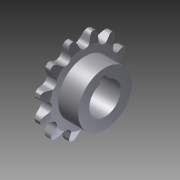
# Autodesk Inventor part: 12t #25 sprocket
Saved by Autodesk Inventor 2012 (Build 160160000, 160)
## iProperties
Created: 2013-07-14
Part Number: 12t #25 sprocket
Material: Default
Document SubType Name: Modeling
Designer: Bryce
Density: 1 g/cm^3
Author: Bryce
Autodesk Inventor part; units mm, degrees
ref_plane "YZ Plane" through (0, 0, 0) normal (1, 0, 0) x (0, 1, 0)
ref_plane "XZ Plane" through (0, 0, 0) normal (0, 1, 0) x (-1, 0, 0)
ref_plane "XY Plane" through (0, 0, 0) normal (0, 0, 1) x (1, 0, 0)
sketch "Sketch1" plane through (0, 0, 0) normal (0, 0, 1) x (1, 0, 0)
  line L0 (0, 0) -> (3.175, 0)
  line L1 (3.175, 0) -> (3.175, 6.1227)
  line L2 (3.175, 8.97) -> (2.4121, 8.97) construction
  line L3 (0, 8.97) -> (0, 6.1227) construction
  line L4 (3.175, 0) -> (9.525, 0)
  line L5 (9.525, 0) -> (9.525, 3.5)
  line L6 (9.525, 3.5) -> (3.175, 3.5)
  line L7 (3.175, 3.5) -> (3.175, 0)
  line L8 (0, -5) -> (9.525, -5) construction
  line L9 (0.7629, 8.97) -> (0, 6.1227)
  line L10 (2.4121, 8.97) -> (3.175, 6.1227)
  line L11 (0.7629, 8.97) -> (0, 8.97) construction
  line L12 (2.4121, 8.97) -> (0.7629, 8.97)
  line L13 (0, 6.1227) -> (0, 0)
  line L14 (3.175, 6.1227) -> (3.175, 8.97) construction
  dimension "d0" = 3.175
  dimension "d1" = 5
  dimension "d3" = 13.97
  dimension "d4" = 8.5
  dimension "d12" = 6.35
  dimension "d26" = 30
  dimension "d27" = 1.6491
  constraints: 30 end point, 9 parallel, 4 perpendicular, 2 horizontal, 1 collinear, 1 horizontal alignment, 1 vertical alignment
  measures "d0" distance of L0.start L0.end
  measures "d1" distance between parallel lines of L4 L8
  measures "d3" distance between parallel lines of L2 L8
  measures "d4" distance between parallel lines of L8 L6
  measures "d12" distance of L0.end L4.end
  measures "d26" angle of L10 L9
  measures "d27" distance of L2.end L9.start
revolve "Revolution1" add sketch "Sketch1" angle 360 about axis through (0, -5, 0) along (1, 0, 0)
sketch "Sketch3" plane through (0, -5, 0) normal (-1, 0, 0) x (0, 0, 1)
  circle A0 centre (0, 0) radius 11.1227 projected
  arc A1 (4.5327, 11.9915) -> (4.0726, 13.3632) centre (2.8057, 12.1753) ccw
  arc A2 (3.1546, 13.6092) -> (2.0703, 12.6513) centre (3.6578, 11.947) ccw
  line L0 (4.4067, 10.8076) -> (4.5327, 11.9915)
  line L1 (1.5875, 11.5629) -> (2.0703, 12.6513)
  arc A3 (-1.5875, 11.5629) -> (1.5875, 11.5629) centre (0, 12.2673) ccw
  line L2 (-1.5875, 11.5629) -> (-2.0703, 12.6513)
  arc A4 (3.1546, 13.6092) -> (-3.1546, 13.6092) centre (0, 0) ccw construction
  arc A5 (-2.0703, 12.6513) -> (-3.1546, 13.6092) centre (-3.6578, 11.947) ccw
  circle A6 centre (0, 0) radius 13.97
  arc A7 (4.0726, 13.3632) -> (3.1546, 13.6092) centre (0, 0) ccw
  arc A8 (-3.1546, 13.6092) -> (-4.0726, 13.3632) centre (0, 0) ccw
  line L3 (-4.4067, 10.8076) -> (-4.5327, 11.9915)
  arc A9 (-4.0726, 13.3632) -> (-4.5327, 11.9915) centre (-2.8057, 12.1753) ccw
  arc A10 (-7.1563, 9.2201) -> (-4.4067, 10.8076) centre (-6.1336, 10.6238) ccw
  arc A11 (-4.0726, 13.3632) -> (-9.5365, 10.2086) centre (0, 0) ccw construction
  line L4 (-7.1563, 9.2201) -> (-8.1186, 9.9211)
  arc A12 (-8.1186, 9.9211) -> (-9.5365, 10.2086) centre (-9.1413, 8.5174) ccw
  arc A13 (-9.5365, 10.2086) -> (-10.2086, 9.5365) centre (0, 0) ccw
  arc A14 (-10.2086, 9.5365) -> (-9.9211, 8.1186) centre (-8.5174, 9.1413) ccw
  arc A15 (-10.8076, 4.4067) -> (-9.2201, 7.1563) centre (-10.6238, 6.1336) ccw
  line L5 (-10.8076, 4.4067) -> (-11.9915, 4.5327)
  arc A16 (-10.2086, 9.5365) -> (-13.3632, 4.0726) centre (0, 0) ccw construction
  arc A17 (-11.9915, 4.5327) -> (-13.3632, 4.0726) centre (-12.1753, 2.8057) ccw
  arc A18 (-13.3632, 4.0726) -> (-13.6092, 3.1546) centre (0, 0) ccw
  line L6 (-9.2201, 7.1563) -> (-9.9211, 8.1186)
  line L7 (-4.4067, -10.8076) -> (-4.5327, -11.9915)
  arc A19 (-4.5327, -11.9915) -> (-4.0726, -13.3632) centre (-2.8057, -12.1753) ccw
  arc A20 (-4.0726, -13.3632) -> (-3.1546, -13.6092) centre (0, 0) ccw
  arc A21 (-9.5365, -10.2086) -> (-4.0726, -13.3632) centre (0, 0) ccw construction
  arc A22 (4.0726, -13.3632) -> (9.5365, -10.2086) centre (0, 0) ccw construction
  arc A23 (7.1563, -9.2201) -> (4.4067, -10.8076) centre (6.1336, -10.6238) ccw
  line L8 (7.1563, -9.2201) -> (8.1186, -9.9211)
  arc A24 (8.1186, -9.9211) -> (9.5365, -10.2086) centre (9.1413, -8.5174) ccw
  arc A25 (9.5365, -10.2086) -> (10.2086, -9.5365) centre (0, 0) ccw
  arc A26 (10.2086, -9.5365) -> (9.9211, -8.1186) centre (8.5174, -9.1413) ccw
  line L9 (9.2201, -7.1563) -> (9.9211, -8.1186)
  arc A27 (10.8076, -4.4067) -> (9.2201, -7.1563) centre (10.6238, -6.1336) ccw
  arc A28 (10.2086, -9.5365) -> (13.3632, -4.0726) centre (0, 0) ccw construction
  arc A29 (11.9915, -4.5327) -> (13.3632, -4.0726) centre (12.1753, -2.8057) ccw
  line L10 (10.8076, -4.4067) -> (11.9915, -4.5327)
  arc A30 (-9.5365, -10.2086) -> (-8.1186, -9.9211) centre (-9.1413, -8.5174) ccw
  line L11 (-7.1563, -9.2201) -> (-8.1186, -9.9211)
  arc A31 (-10.2086, -9.5365) -> (-9.5365, -10.2086) centre (0, 0) ccw
  arc A32 (-9.9211, -8.1186) -> (-10.2086, -9.5365) centre (-8.5174, -9.1413) ccw
  line L12 (-9.2201, -7.1563) -> (-9.9211, -8.1186)
  arc A33 (-9.2201, -7.1563) -> (-10.8076, -4.4067) centre (-10.6238, -6.1336) ccw
  line L13 (-10.8076, -4.4067) -> (-11.9915, -4.5327)
  arc A34 (-13.3632, -4.0726) -> (-11.9915, -4.5327) centre (-12.1753, -2.8057) ccw
  arc A35 (-13.3632, -4.0726) -> (-10.2086, -9.5365) centre (0, 0) ccw construction
  arc A36 (-13.6092, -3.1546) -> (-13.3632, -4.0726) centre (0, 0) ccw
  arc A37 (-4.4067, -10.8076) -> (-7.1563, -9.2201) centre (-6.1336, -10.6238) ccw
  arc A38 (11.5629, 1.5875) -> (11.5629, -1.5875) centre (12.2673, 0) ccw
  line L14 (11.5629, 1.5875) -> (12.6513, 2.0703)
  arc A39 (12.6513, 2.0703) -> (13.6092, 3.1546) centre (11.947, 3.6578) ccw
  line L15 (10.8076, 4.4067) -> (11.9915, 4.5327)
  arc A40 (13.3632, 4.0726) -> (11.9915, 4.5327) centre (12.1753, 2.8057) ccw
  arc A41 (13.6092, 3.1546) -> (13.3632, 4.0726) centre (0, 0) ccw
  line L16 (11.5629, -1.5875) -> (12.6513, -2.0703)
  arc A42 (13.6092, -3.1546) -> (12.6513, -2.0703) centre (11.947, -3.6578) ccw
  arc A43 (13.6092, -3.1546) -> (13.6092, 3.1546) centre (0, 0) ccw construction
  arc A44 (13.3632, -4.0726) -> (13.6092, -3.1546) centre (0, 0) ccw
  arc A45 (9.2201, 7.1563) -> (10.8076, 4.4067) centre (10.6238, 6.1336) ccw
  arc A46 (13.3632, 4.0726) -> (10.2086, 9.5365) centre (0, 0) ccw construction
  line L17 (9.2201, 7.1563) -> (9.9211, 8.1186)
  arc A47 (9.9211, 8.1186) -> (10.2086, 9.5365) centre (8.5174, 9.1413) ccw
  arc A48 (10.2086, 9.5365) -> (9.5365, 10.2086) centre (0, 0) ccw
  arc A49 (9.5365, 10.2086) -> (8.1186, 9.9211) centre (9.1413, 8.5174) ccw
  line L18 (7.1563, 9.2201) -> (8.1186, 9.9211)
  arc A50 (4.4067, 10.8076) -> (7.1563, 9.2201) centre (6.1336, 10.6238) ccw
  arc A51 (9.5365, 10.2086) -> (4.0726, 13.3632) centre (0, 0) ccw construction
  arc A52 (1.5875, -11.5629) -> (-1.5875, -11.5629) centre (0, -12.2673) ccw
  line L19 (1.5875, -11.5629) -> (2.0703, -12.6513)
  arc A53 (2.0703, -12.6513) -> (3.1546, -13.6092) centre (3.6578, -11.947) ccw
  line L20 (-1.5875, -11.5629) -> (-2.0703, -12.6513)
  line L21 (4.4067, -10.8076) -> (4.5327, -11.9915)
  arc A54 (3.1546, -13.6092) -> (4.0726, -13.3632) centre (0, 0) ccw
  arc A55 (-3.1546, -13.6092) -> (-2.0703, -12.6513) centre (-3.6578, -11.947) ccw
  arc A56 (-3.1546, -13.6092) -> (3.1546, -13.6092) centre (0, 0) ccw construction
  arc A57 (4.0726, -13.3632) -> (4.5327, -11.9915) centre (2.8057, -12.1753) ccw
  line L22 (-11.5629, 1.5875) -> (-12.6513, 2.0703)
  arc A58 (-11.5629, -1.5875) -> (-11.5629, 1.5875) centre (-12.2673, 0) ccw
  line L23 (-11.5629, -1.5875) -> (-12.6513, -2.0703)
  arc A59 (-12.6513, -2.0703) -> (-13.6092, -3.1546) centre (-11.947, -3.6578) ccw
  arc A60 (-13.6092, 3.1546) -> (-13.6092, -3.1546) centre (0, 0) ccw construction
  arc A61 (-13.6092, 3.1546) -> (-12.6513, 2.0703) centre (-11.947, 3.6578) ccw
  arc A62 (-4.4511, 10.1932) -> (-6.602, 8.9514) centre (0, 0) ccw
  arc A63 (1.2418, 11.0532) -> (-1.2418, 11.0532) centre (0, 0) ccw
  arc A64 (6.602, 8.9514) -> (4.4511, 10.1932) centre (0, 0) ccw
  arc A65 (10.1932, 4.4511) -> (8.9514, 6.602) centre (0, 0) ccw
  arc A66 (11.0532, -1.2418) -> (11.0532, 1.2418) centre (0, 0) ccw
  arc A67 (8.9514, -6.602) -> (10.1932, -4.4511) centre (0, 0) ccw
  arc A68 (4.4511, -10.1932) -> (6.602, -8.9514) centre (0, 0) ccw
  arc A69 (-1.2418, -11.0532) -> (1.2418, -11.0532) centre (0, 0) ccw
  arc A70 (-6.602, -8.9514) -> (-4.4511, -10.1932) centre (0, 0) ccw
  arc A71 (-10.1932, -4.4511) -> (-8.9514, -6.602) centre (0, 0) ccw
  arc A72 (-11.0532, 1.2418) -> (-11.0532, -1.2418) centre (0, 0) ccw
  arc A73 (-8.9514, 6.602) -> (-10.1932, 4.4511) centre (0, 0) ccw
  circle A74 centre (0, 0) radius 5 projected
  line L24 (-1.5875, 3.4125) -> (1.5875, 3.4125)
  line L25 (1.5875, 3.4125) -> (1.5875, 6.5875)
  line L26 (1.5875, 6.5875) -> (-1.5875, 6.5875)
  line L27 (-1.5875, 6.5875) -> (-1.5875, 3.4125)
  point P0 (0, 5)
  dimension "d44" = 10
  dimension "d30" = 1.7367
  dimension "d31" = 12.2673
  dimension "d32" = 1.1906
  dimension "d33" = 1.7367
  dimension "d34" = 3.175
  dimension "d35" = 360
  dimension "d36" = 6.35
  dimension "d37" = 13.97
  dimension "d38" = 27.94
  dimension "d41" = 3.175
  dimension "d42" = 3.175
  dimension "d43" = 1.5875
  dimension "d45" = 6.5875
  constraints: 168 point on circle, 73 centre point, 56 end point, 13 coincident, 4 tangent, 2 horizontal alignment, 2 parallel, 2 vertical alignment, 1 equal length, 1 equal radius, 1 horizontal, 1 perpendicular, 190 other
  measures "d30" radius of A3
  measures "d31" distance of A6.centre A3.centre
  measures "d32" distance of L2.start L2.end
  measures "d33" radius of A5
  measures "d34" distance of L1.start L2.start
  measures "d36" distance of A50.centre A3.centre
  measures "d37" radius of A51
  measures "d38" diameter of A6
  measures "d41" distance of L25.end L26.end
  measures "d42" distance of L24.end L25.end
  measures "d43" distance from line of point (0, 0) L25
  measures "d45" distance from line of A63.centre L26
extrude "Extrusion2" cut sketch "Sketch3" against normal through all contours A0 A38 | A0 A38 L14 A39 A6 A42 L16 | A45 A0 | A0 A45 L17 A47 A6 A40 L15 | A27 L10 A29 A6 A26 L9 A0 | A0 A27 | A50 A0 | A0 A50 L0 A1 A6 A49 L18 | A23 L8 A24 A6 A57 L21 A0 | A0 A23 | A3 A0 | A0 A3 L2 A5 A6 A2 L1 | A52 L19 A53 A6 A55 L20 A0 | A0 A52 | A10 A0 | A0 A10 L4 A12 A6 A9 L3 | A37 L7 A19 A6 A30 L11 A0 | A0 A37 | A15 A0 | A0 A15 L5 A17 A6 A14 L6 | A33 L12 A32 A6 A34 L13 A0 | A0 A33 | A58 A0 | A0 A58 L23 A59 A6 A61 L22
extrude "Extrusion3" cut sketch "Sketch3" against normal through all contours L25 L24 L27 A74 | A74 L27 L26 L25 picked at (0.1791, 3.932)
equation "\"d33\" = d30"
equation "\"d38\" = 2 * d37"
equation "\"d43\" = 0.5 * d41"
equation "\"d45\" = 0.5 * d44 + d43"
body "Solid1"
